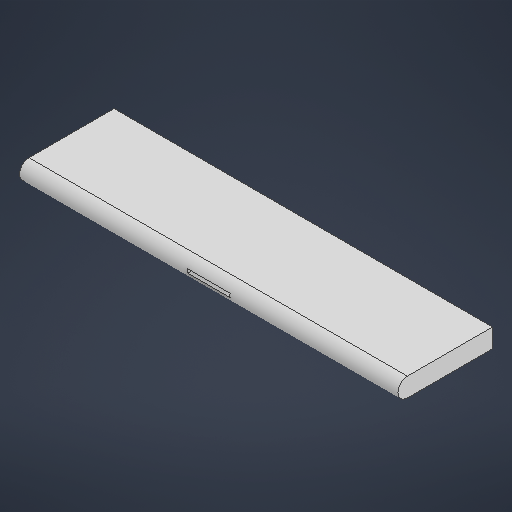
# Autodesk Inventor part: RCPlaneElevator
Saved by Autodesk Inventor 2026.1 (Build 301233000, 233)
## iProperties
Created: 2026-03-17
Part Number: RCPlaneElevator
Material: Generic
Document SubType Name: Modeling
Designer: morri
Density: 1 g/cm^3
Appearance: Default
Author: morri
Autodesk Inventor part; units mm, degrees
ref_plane "YZ Plane" through (0, 0, 0) normal (1, 0, 0) x (0, 1, 0)
ref_plane "XZ Plane" through (0, 0, 0) normal (0, 1, 0) x (-1, 0, 0)
ref_plane "XY Plane" through (0, 0, 0) normal (0, 0, 1) x (1, 0, 0)
sketch "Sketch2" plane through (0, 0, 0) normal (0, 1, 0) x (-1, 0, 0)
  line L0 (0, 0) -> (-100, 0)
  line L1 (-100, 0) -> (-100, 25)
  line L2 (-100, 25) -> (0, 25)
  line L3 (0, 25) -> (0, 0)
  dimension "d10" = 100
  dimension "d11" = 25
  constraints: 8 end point, 2 parallel, 1 horizontal, 1 perpendicular
  measures "d10" distance of L1.end L2.end
  measures "d11" distance of L0.end L1.end
extrude "Extrusion2" add sketch "Sketch2" along normal blind 5
sketch "Sketch3" plane through (0, 0, 25) normal (0, 0, 1) x (1, 0, 0)
  line L0 (0, 0) -> (100, 0) construction
  line L1 (0, 0) -> (44.4, 0) construction
  line L2 (44.4, 0) -> (44.4, 2) construction
  line L3 (44.4, 2) -> (0, 2) construction
  line L4 (0, 2) -> (0, 0) construction
  line L5 (44.4, 2) -> (55.6, 2)
  line L6 (55.6, 2) -> (55.6, 3)
  line L7 (55.6, 3) -> (44.4, 3)
  line L8 (44.4, 3) -> (44.4, 2)
  dimension "d14" = 44.4
  dimension "d15" = 2
  dimension "d16" = 11.2
  dimension "d17" = 1
  constraints: 16 end point, 4 parallel, 2 horizontal, 2 perpendicular
  measures "d14" distance of L3.end L2.end
  measures "d15" distance of L2.end L1.end
  measures "d16" distance of L7.end L6.end
  measures "d17" distance of L6.end L5.end
extrude "Extrusion3" cut sketch "Sketch3" against normal blind 12.5
fillet "Fillet2" radius 2.5 2 edges at (50, 5, 25) (50, 0, 25)
shell "Shell1" thickness 1 removed faces 0
body "Solid2"
